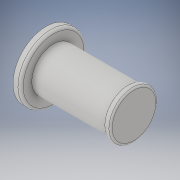
# Autodesk Inventor part: Connector_pin_base
Saved by Autodesk Inventor 2019.3 (Build 233278000, 278)
## iProperties
Created: 2019-02-01
Part Number: Connector_pin_base
Material: Generic
Document SubType Name: Modeling
Designer: Varga Daniel
Density: 1 g/cm^3
Appearance: Default
Author: Varga Daniel
Autodesk Inventor part; units mm, degrees
ref_plane "YZ Plane" through (0, 0, 0) normal (1, 0, 0) x (0, 1, 0)
ref_plane "XZ Plane" through (0, 0, 0) normal (0, 1, 0) x (-1, 0, 0)
ref_plane "XY Plane" through (0, 0, 0) normal (0, 0, 1) x (1, 0, 0)
sketch "Sketch1" plane through (0, 0, 0) normal (0, 0, 1) x (1, 0, 0)
  line L0 (0, 0) -> (9.0624, 0) construction
  line L1 (0, 0) -> (0, 6.22) construction
  line L2 (0, 3.75) -> (0.563, 3.75)
  line L3 (0.863, 3.45) -> (0.863, 2.475)
  line L4 (0.863, 2.475) -> (9.988, 2.475)
  line L5 (9.988, 2.475) -> (9.988, 0)
  line L6 (0, 0) -> (0, 3.75)
  line L7 (0, 0) -> (9.988, 0)
  line L8 (9.288, 2.475) -> (9.288, 2.6)
  line L9 (9.988, 2.475) -> (9.988, 2.4774)
  arc A0 (9.988, 2.4774) -> (9.8454, 2.7031) centre (9.738, 2.4774) ccw
  arc A1 (9.8454, 2.7031) -> (9.288, 2.6) centre (9.6379, 2.267) ccw
  line L10 (9.8454, 2.7031) -> (9.8454, -0.0362) construction
  line L11 (8.9584, 2.75) -> (10.3858, 2.75) construction
  arc A2 (0.863, 3.45) -> (0.563, 3.75) centre (0.563, 3.45) ccw
  line L12 (0.863, 2.475) -> (0.863, 0)
  dimension "d0" = 1.726
  dimension "d1" = 7.5
  dimension "d2" = 4.95
  dimension "d3" = 19.976
  dimension "d4" = 0.25
  dimension "d5" = 8.425
  dimension "d6" = 0.483
  dimension "d7" = 0.125
  dimension "d10" = 5.5
  dimension "d11" = 0.275
  dimension "d12" = 0.7
  dimension "d13" = 0.3
  constraints: 26 end point, 6 point on circle, 5 perpendicular, 5 tangent, 4 point on line, 3 centre point, 3 horizontal, 3 vertical, 2 collinear, 1 coincident
  measures "d0" diameter of L3 L1
  measures "d1" diameter of L2 L0
  measures "d2" diameter of L4 L0
  measures "d3" diameter of L5 L1
  measures "d4" radius of A0
  measures "d5" distance between parallel lines of L8 L3
  measures "d6" radius of A1
  measures "d7" distance from line of L8.end L4
  measures "d10" diameter of L11 L0
  measures "d11" distance between parallel lines of L11 L4
  measures "d12" distance between parallel lines of L8 L5
  measures "d13" radius of A2
revolve "Revolution1" add sketch "Sketch1" angle 360 about axis through (0, 0, 0) along (1, 0, 0)
equation "\"d0\" = Collar_thickness"
equation "\"d1\" = Collar_diameter"
equation "\"d2\" = Pin_diameter"
equation "\"d3\" = Pin_overall_length"
equation "\"d5\" = Pin_inner_length"
equation "\"d10\" = Upper_ring_diameter"
equation "\"Collar_thickness\" = 1.726"
equation "\"Pin_diameter\" = 4.95"
equation "\"Collar_diameter\" = 7.5"
equation "\"Pin_overall_length\" = 19.976"
equation "\"Pin_inner_length\" = 8.425"
equation "\"Upper_ring_diameter\" = 5.5"
body "Solid1"
